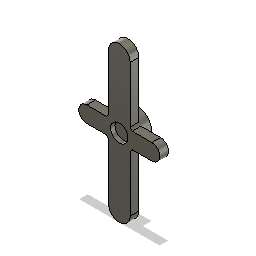
section_controle v39 (Autodesk Fusion 360 archive; units mm, degrees)
design "servo_arm_att"
Autodesk Fusion 360 part; units mm, degrees
sketch "Esquisse1" plane through (0, 0, 0) normal (0, 1, 0) x (1, 0, 0)
  circle A0 centre (0, 0) radius 35
  dimension "d1" = 70
  constraint coincident A0.centre origin
  measures "d1" diameter of A0
sketch "Esquisse2" plane through (0, 0, 0) normal (0, 1, 0) x (1, 0, 0)
  circle A0 centre (0, 0) radius 32.5
  circle A1 centre (0, 0) radius 35
  dimension "d2" = 65
  dimension "d3" = 70
  constraint coincident A0.centre A1.centre
  measures "d2" diameter of A0
  measures "d3" diameter of A1
sketch "Esquisse3" plane through (0, 0, 35.4) normal (0, 0, 1) x (1, 0, 0)
  circle A0 centre (0, 5.75) radius 5.75
  circle A1 centre (0, 5.75) radius 5.75 construction
  circle A2 centre (0, 5.75) radius 3.5
  circle A3 centre (0, 5.75) radius 3
  dimension "d6" = 7
  dimension "d7" = 6
  constraint concentric A0 A1
  constraint concentric A1 A2
  constraint concentric A2 A3
  measures "d6" diameter of A2
  measures "d7" diameter of A3
extrude "Extrusion2" add sketch "Esquisse3" along normal blind 2 contours A2 makes body 1
sketch "Esquisse4" plane through (0, 0, 37.4) normal (0, 0, 1) x (1, 0, 0)
  circle A0 centre (0, 5.75) radius 3
  circle A1 centre (0, 5.75) radius 3.5
  line L0 (0, 5.75) -> (0, 23.6) construction
  line L1 (0, 5.75) -> (0, -12.1) construction
  line L2 (0, 23.6) -> (6, 23.6) construction
  line L3 (0, 23.6) -> (-6, 23.6) construction
  line L4 (0, 5.75) -> (-2.5, 5.75)
  line L5 (-2.5, 5.75) -> (-2.5, 23.6)
  line L6 (-2.5, 23.6) -> (0, 23.6)
  line L7 (0, 23.6) -> (0, 5.75)
  line L8 (0, 5.75) -> (2.5, 5.75)
  line L9 (0, 23.6) -> (0, 5.75)
  line L10 (2.5, 5.75) -> (2.5, 23.6)
  line L11 (2.5, 23.6) -> (0, 23.6)
  line L12 (-2.5, 5.75) -> (-2.5, -12.1)
  line L13 (-2.5, -12.1) -> (0, -12.1)
  line L14 (2.5, -12.1) -> (0, -12.1)
  line L15 (2.5, 5.75) -> (2.5, -12.1)
  line L16 (0, 5.75) -> (2.5, 5.75)
  line L17 (0, 5.75) -> (-2.5, 5.75)
  line L18 (0, -12.1) -> (0, 5.75)
  line L19 (0, 5.75) -> (-9.35, 5.75) construction
  line L20 (0, 5.75) -> (9.35, 5.75) construction
  line L21 (-9.35, 5.75) -> (-9.35, 6) construction
  line L22 (-9.35, 6) -> (-9.35, 10) construction
  line L23 (-9.35, 5.75) -> (-9.35, 1.75) construction
  line L24 (9.35, 6) -> (9.35, 10) construction
  line L25 (9.35, 5.75) -> (9.35, 1.75) construction
  line L26 (0, 5.75) -> (-9.35, 5.75)
  line L27 (-9.35, 5.75) -> (-9.35, 3.9)
  line L28 (-9.35, 3.9) -> (0, 3.9)
  line L29 (0, 3.9) -> (0, 5.75)
  line L30 (-9.35, 7.6) -> (0, 7.6)
  line L31 (-9.35, 5.75) -> (-9.35, 7.6)
  line L32 (9.35, 7.6) -> (0, 7.6)
  line L33 (9.35, 5.75) -> (9.35, 7.6)
  line L34 (9.35, 5.75) -> (9.35, 3.9)
  line L35 (9.35, 3.9) -> (0, 3.9)
  line L36 (0, 5.75) -> (9.35, 5.75)
  dimension "d10" = 17.85
  dimension "d11" = 17.85
  dimension "d12" = 2.5
  dimension "d13" = 9.35
  dimension "d14" = 9.35
  dimension "d15" = 4
  dimension "d16" = 1.85
  constraint coincident A0.centre A1.centre
  constraint vertical L0
  constraint parallel L0 L1
  constraint perpendicular L0 L2
  constraint perpendicular L0 L3
  constraint horizontal L4
  constraint vertical L5
  constraint horizontal L6
  constraint vertical L7
  constraint coincident L3 L5.end
  constraint symmetric A0.centre L7 A1.centre
  constraint symmetric L4.end L7 L8.end
  constraint symmetric L5.end L7 L10.end
  constraint symmetric L0.end L7 L2.start
  constraint symmetric A0.centre L8 A1.centre
  constraint symmetric L4.end L8 L5.start
  constraint symmetric L5.end L8 L12.end
  constraint symmetric L0.end L8 L1.end
  constraint symmetric L10.start L8 L15.start
  constraint symmetric L8 L0.end L1.end
  constraint symmetric L8 L10.end L14.start
  constraint perpendicular L1 L19
  constraint perpendicular L1 L20
  constraint perpendicular L19 L21
  constraint perpendicular L19 L22
  constraint perpendicular L19 L23
  constraint symmetric L9 L19.end L20.end
  constraint symmetric L9 L21.end L24.start
  constraint symmetric L9 L22.end L24.end
  constraint symmetric L9 L23.end L25.end
  constraint horizontal L26
  constraint vertical L27
  constraint horizontal L28
  constraint vertical L29
  constraint coincident L23 L27.end
  constraint symmetric L19.end L26 L21.start
  constraint symmetric L27.end L26 L30.start
  constraint symmetric L28.end L26 L30.end
  constraint symmetric A0.centre L9 A1.centre
  constraint symmetric L9 L27.end L34.end
  constraint symmetric L9 L28.end L29.start
  constraint symmetric L9 L30.start L32.start
  constraint symmetric L9 L30.end L32.end
  measures "d10" distance of A0.centre L0.end
  measures "d11" distance of A0.centre L1.end
  measures "d12" distance of A0.centre L4.end
  measures "d13" distance of A0.centre L19.end
  measures "d14" distance of A0.centre L20.end
  measures "d15" distance of L19.end L23.end
  measures "d16" distance of A0.centre L28.end
extrude "Extrusion3" add sketch "Esquisse4" along normal blind 2 bodies 1
fillet "Congé1" radius 2.5 4 edges at (-2.5, 23.6, 38.4) (2.5, 23.6, 38.4) (-2.5, -12.1, 38.4) (2.5, -12.1, 38.4) on bodies 1
fillet "Congé2" radius 1.85 4 edges at (-9.35, 7.6, 38.4) (-9.35, 3.9, 38.4) (9.35, 7.6, 38.4) (9.35, 3.9, 38.4) on bodies 1
sketch "Esquisse6" plane through (0, 0, 39.4) normal (0, 0, 1) x (1, 0, 0)
  arc A0 (7.5, 3.9) -> (7.5, 7.6) centre (7.5, 5.75) ccw
  line L0 (7.5, 7.6) -> (2.9711, 7.6)
  arc A1 (2.9711, 7.6) -> (2.5, 8.1995) centre (0, 5.75) ccw
  line L1 (2.5, 8.1995) -> (2.5, 21.1)
  arc A2 (2.5, 21.1) -> (-2.5, 21.1) centre (0, 21.1) ccw
  line L2 (-2.5, 21.1) -> (-2.5, 8.1995)
  arc A3 (-2.5, 8.1995) -> (-2.9711, 7.6) centre (0, 5.75) ccw
  line L3 (-2.9711, 7.6) -> (-7.5, 7.6)
  arc A4 (-7.5, 7.6) -> (-7.5, 3.9) centre (-7.5, 5.75) ccw
  line L4 (-7.5, 3.9) -> (-2.9711, 3.9)
  arc A5 (-2.9711, 3.9) -> (-2.5, 3.3005) centre (0, 5.75) ccw
  line L5 (-2.5, 3.3005) -> (-2.5, -9.6)
  arc A6 (-2.5, -9.6) -> (2.5, -9.6) centre (0, -9.6) ccw
  line L6 (2.5, -9.6) -> (2.5, 3.3005)
  arc A7 (2.5, 3.3005) -> (2.9711, 3.9) centre (0, 5.75) ccw
  line L7 (2.9711, 3.9) -> (7.5, 3.9)
  circle A8 centre (0, 5.75) radius 2
  dimension "d23" = 4
  constraint concentric A1 A8
  measures "d23" diameter of A8
extrude "Extrusion4" cut sketch "Esquisse6" against normal blind 1 contours A8 bodies 1
copy_body "Corps->Comp1" bodies 1 removing the originals makes body 2 in component "servo_arm"
component "servo_arm" placed x (1, 0, 0) y (0, 1, 0) z (0, 0, 1) at (0, 0, 0)
equation "d10 = ( 35.7 / 2 ) * 1 mm"
equation "d11 = ( 35.7 / 2 ) * 1 mm"
equation "d13 = ( 18.7 / 2 ) * 1 mm"
equation "d14 = ( 18.7 / 2 ) * 1 mm"
equation "d16 = ( 3.7 / 2 ) * 1 mm"
named bodies: "servo_arm"
